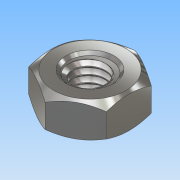
# Autodesk Inventor part: м3 гайка
Saved by Autodesk Inventor 2017 (Build 210142000, 142)
## iProperties
Part Number: м3 гайка
Material: Типовые
Document SubType Name: Modeling
Designer: STALKER
Density: 1 g/cm^3
Appearance: Хром - полированный
Author: STALKER
Autodesk Inventor part; units mm, degrees
ref_plane "YZ Plane" through (0, 0, 0) normal (1, 0, 0) x (0, 1, 0)
ref_plane "XZ Plane" through (0, 0, 0) normal (0, 1, 0) x (-1, 0, 0)
ref_plane "XY Plane" through (0, 0, 0) normal (0, 0, 1) x (1, 0, 0)
sketch "Эскиз1" plane through (0, 0, 0) normal (0, 0, 1) x (1, 0, 0)
  line L0 (0, 3.1754) -> (2.75, 1.5877)
  line L1 (2.75, 1.5877) -> (2.75, -1.5877)
  line L2 (2.75, -1.5877) -> (0, -3.1754)
  line L3 (0, -3.1754) -> (-2.75, -1.5877)
  line L4 (-2.75, -1.5877) -> (-2.75, 1.5877)
  line L5 (-2.75, 1.5877) -> (0, 3.1754)
  circle A0 centre (0, 0) radius 1.5
  dimension "d0" = 5.5
  dimension "d1" = 3
  constraints: 12 end point, 2 coincident, 1 centre point, 13 other
  measures "d0" distance between parallel lines of L1 L4
  measures "d1" diameter of A0
extrude "Выдавливание1" add sketch "Эскиз1" along normal mid plane 2.5
chamfer "Фаска1" distance 0.2 angle 45 2 edges at (-1.5, 0, 1.25) (-1.5, 0, -1.25)
sketch "Эскиз4" plane through (0, 0, 0) normal (1, 0, 0) x (0, 1, 0)
  line L0 (3.5759, 0.564) -> (1.5391, 1.9396)
  line L1 (1.5391, 1.9396) -> (6.9458, 1.9396)
  line L2 (6.9458, 1.9396) -> (6.9458, -1.9396)
  line L3 (6.9458, -1.9396) -> (1.5391, -1.9396)
  line L4 (1.5391, -1.9396) -> (3.5759, -0.564)
  line L5 (0, 0) -> (8, 0) construction
  line L6 (1.5391, 1.9396) -> (1.5391, -1.9396) construction
  line L7 (0, 0) -> (0, 12) construction
  line L8 (3.5759, 0.564) -> (3.5759, -0.564)
  constraints: 18 end point, 2 horizontal, 2 perpendicular, 2 vertical, 1 other
revolve "Вращение2" cut sketch "Эскиз4" angle 360 about axis through (0, 0, 0) along (0, 0, 1)
thread "Резьба2" size "M3x0.5" class "6H" standard "ANSI Metric M Profile" full length
sketch "Эскиз6" plane through (0, 0, 1.05) normal (-1, 0, 0) x (0, 1, 0)
  line L0 (1.5, 0) -> (1.5, 2.1)
  line L1 (1.5, 2.1) -> (1.1293, 2.1)
  line L2 (1.1293, 2.1) -> (1.1293, 0)
  line L3 (1.1293, 0) -> (1.5, 0)
  line L4 (0, -1.1385) -> (0, 3.0138) projected
  constraints: 8 end point
revolve "Вращение3" add sketch "Эскиз6" angle 360 about axis through (0, 0, 1.05) along (0, 0, -1) separate body
sketch "Эскиз5" plane through (0, 1.5, 1.05) normal (1, 0, 0) x (0, 0, -1)
  line L0 (-0.2918, -0.0255) -> (-0.2501, -0.0255) construction
  line L1 (0.0416, -0.3456) -> (-0.0001, -0.4257) construction
  line L2 (-0.5001, -0.4257) -> (-0.5418, -0.3456) construction
  line L3 (-0.2084, -0.0255) -> (-0.2501, 0.0546) construction
  line L4 (-0.2501, 0.0546) -> (-0.2918, -0.0255) construction
  line L5 (-0.5001, -0.4257) -> (-0.4584, -0.3456) construction
  line L6 (-0.2084, -0.0255) -> (-0.0418, -0.3456)
  line L7 (-0.5418, -0.3456) -> (-0.4584, -0.3456) construction
  arc A0 (-0.5418, -0.3456) -> (-0.5001, -0.3709) centre (-0.5001, -0.3239) ccw construction
  line L8 (0.0416, -0.3456) -> (-0.0418, -0.3456) construction
  line L9 (-0.5001, -0.4257) -> (-0.5001, -0.3456) construction
  line L10 (-0.0001, -0.4257) -> (-0.0001, -0.3456) construction
  line L11 (-0.2501, 0.0546) -> (-0.2501, -0.0002) construction
  line L12 (-0.5001, -0.3709) -> (-0.0001, -0.3709)
  arc A1 (-0.5001, -0.3709) -> (-0.4584, -0.3456) centre (-0.5001, -0.3239) ccw
  line L13 (-0.0418, -0.3456) -> (-0.0001, -0.4257) construction
  line L14 (-0.4584, -0.3456) -> (-0.2918, -0.0255)
  line L15 (-0.0001, -0.0002) -> (-0.0001, 0.0177)
  line L16 (-0.0001, 0.0177) -> (-0.0001, -0.0002)
  line L17 (-0.0001, -0.0002) -> (0.0334, -0.0002)
  arc A2 (-0.0418, -0.3456) -> (-0.0001, -0.3709) centre (-0.0001, -0.3239) ccw
  arc A3 (-0.0001, -0.3709) -> (0.0416, -0.3456) centre (-0.0001, -0.3239) ccw construction
  arc A4 (-0.2501, -0.0002) -> (-0.2918, -0.0255) centre (-0.2501, -0.0471) ccw
  arc A5 (-0.2084, -0.0255) -> (-0.2501, -0.0002) centre (-0.2501, -0.0471) ccw
  line L18 (-0.2501, -0.0002) -> (-0.2501, -0.0255) construction
  line L19 (-0.2501, -0.0255) -> (-0.2084, -0.0255) construction
  dimension "d30" = 55
  dimension "d31" = 0.08
  dimension "d32" = 0.08
  dimension "Эскиз5_ThreadOffset" = 0
  dimension "Эскиз5_MajorRadius" = 0.3707
  dimension "d35" = 0.5
  dimension "Эскиз5_MinorRadius" = 0
  constraints: 40 end point, 12 point on circle, 10 parallel, 8 tangent, 6 centre point, 6 collinear, 2 midpoint, 2 point on line, 1 horizontal, 1 perpendicular, 3 other
  measures "d30" angle of L6 L14
  measures "d31" distance of L3.end L0.end
  measures "d32" distance of L1.end L10.end
  measures "Эскиз5_ThreadOffset" distance between parallel lines of L15 L10
  measures "Эскиз5_MajorRadius" distance from line of L12 L15.start
  measures "d35" distance from line of L1.end L9
  measures "Эскиз5_MinorRadius" distance edge to line of A5 L17
coil "Пружина2" sketch "Эскиз5" operation cut axis through (0, 0, 1.05) along (0, 0, -1) pitch 0.5005 turns 6.193806 hand right bodies 2
equation "\"d30\" = d37"
equation "\"d31\" = 0.160083 * Эскиз5_Pitch"
equation "\"d32\" = 0.160083 * Эскиз5_Pitch"
equation "\"d35\" = Эскиз5_Pitch"
equation "\"d16\" = 55deg"
equation "\"Эскиз2_Pitch\" = 0.5"
equation "\"d37\" = 55deg"
equation "\"Эскиз5_Pitch\" = 0.5"
